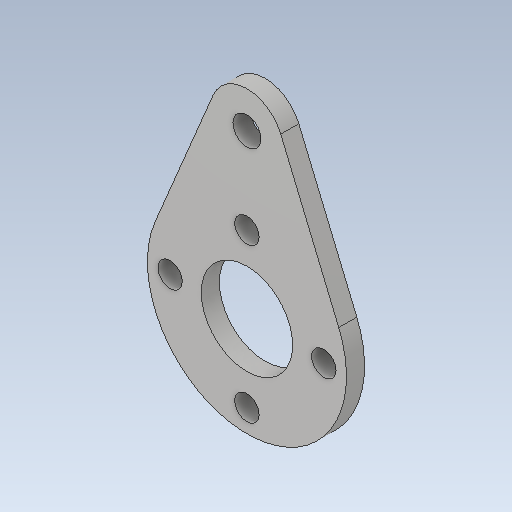
# Autodesk Inventor part: Slider_crank_horn
Saved by Autodesk Inventor 2020.4 (Build 244396000, 396)
## iProperties
Created: 2016-08-24
Part Number: Slider_crank_horn
Material: GFRP
Document SubType Name: Modeling
Designer: hiro
Density: 1.75 g/cm^3
Appearance: 滑らか - 淡い灰色
Mass: 1.33535 g
Surface Area: 10.8308 cm^2
Volume: 0.763059 cm^3
Category: 付け根
Author: hiro
Autodesk Inventor part; units mm, degrees
ref_plane "YZ Plane" through (0, 0, 0) normal (1, 0, 0) x (0, 1, 0)
ref_plane "XZ Plane" through (0, 0, 0) normal (0, 1, 0) x (-1, 0, 0)
ref_plane "XY Plane" through (0, 0, 0) normal (0, 0, 1) x (1, 0, 0)
derived "付け根_基準フレーム_6_1.ipt"
sketch "スケッチ1" plane through (0, 0, 0) normal (0, 0, 1) x (1, 0, 0)
  circle A0 centre (0, 0) radius 11 construction
  circle A1 centre (-13.5, -1) radius 1.35 construction
  line L0 (-13.5, -1) -> (13.5, -1) construction
  line L1 (13.5, -1) -> (13.5, -28) construction
  line L2 (13.5, -28) -> (-13.5, -28) construction
  line L3 (-13.5, -28) -> (-13.5, -1) construction
  circle A2 centre (13.5, -1) radius 1.35 construction
  circle A3 centre (-13.5, -28) radius 1.35 construction
  circle A4 centre (13.5, -28) radius 1.35 construction
  line L4 (0, 18) -> (0, -18) construction
  circle A5 centre (0, -18) radius 7 construction
  line L5 (-12.5, 29.5) -> (-12.5, 24.5) construction
  line L6 (-12.5, 24.5) -> (-7.9564, -18.8342) construction
  line L7 (-12.5, 29.5) -> (12.5, 29.5) construction
  line L8 (12.5, 29.5) -> (12.5, 24.5) construction
  line L9 (12.5, 24.5) -> (7.9564, -18.8342) construction
  arc A6 (-7.9564, -18.8342) -> (7.9564, -18.8342) centre (0, -18) ccw construction
  circle A7 centre (-9.5, 27) radius 1.55 construction
  circle A8 centre (9.5, 27) radius 1.55 construction
  line L10 (-5.51, 27.01) -> (5.51, 27.01) construction
  line L11 (5.51, 27.01) -> (5.51, 24.49) construction
  line L12 (5.51, 24.49) -> (-5.51, 24.49) construction
  line L13 (-5.51, 24.49) -> (-5.51, 27.01) construction
  circle A9 centre (-4.46, 27.01) radius 1.05 construction
  circle A10 centre (-4.46, 24.49) radius 1.05 construction
  circle A11 centre (4.46, 27.01) radius 1.05 construction
  circle A12 centre (4.46, 24.49) radius 1.05 construction
  line L14 (5.5, 27) -> (-5.5, 27) construction
  line L15 (-5.5, 27) -> (-5.5, 24.5) construction
  line L16 (-5.5, 24.5) -> (5.5, 24.5) construction
  line L17 (5.5, 24.5) -> (5.5, 27) construction
  circle A13 centre (0, -18) radius 4.05 construction
  circle A14 centre (0, 8.5) radius 1.35
  circle A15 centre (-8.5, 0) radius 1.35
  circle A16 centre (0, -8.5) radius 1.35
  circle A17 centre (8.5, 0) radius 1.35
  circle A18 centre (0, 0) radius 5.05
  line L18 (-10.147, 4.2472) -> (-3.7359, 19.5638)
  line L19 (3.7359, 19.5638) -> (10.147, 4.2472)
  arc A19 (-10.147, 4.2472) -> (10.147, 4.2472) centre (0, 0) ccw
  arc A20 (3.7359, 19.5638) -> (-3.7359, 19.5638) centre (0, 18) ccw
  circle A21 centre (0, 18) radius 1.55
  line L20 (-10.9545, 1) -> (-14.0575, 1) construction
  line L21 (-14.0575, 1) -> (-24.81, -5.5) construction
  line L22 (-24.81, -5.5) -> (-24.81, -23.5) construction
  line L23 (-24.81, -23.5) -> (-14.0575, -30) construction
  line L24 (-14.0575, -30) -> (14.0575, -30) construction
  line L25 (14.0575, -30) -> (24.81, -23.5) construction
  line L26 (24.81, -23.5) -> (24.81, -5.5) construction
  line L27 (24.81, -5.5) -> (14.0575, 1) construction
  line L28 (14.0575, 1) -> (10.9545, 1) construction
  arc A22 (-10.9545, 1) -> (10.9545, 1) centre (0, 0) ccw construction
  line L29 (-21.76, -10.49) -> (-19.74, -10.49) construction
  line L30 (-19.74, -10.49) -> (-19.74, -18.51) construction
  line L31 (-19.74, -18.51) -> (-21.76, -18.51) construction
  line L32 (-21.76, -18.51) -> (-21.76, -10.49) construction
  line L33 (-19.75, -10.5) -> (-21.75, -10.5) construction
  line L34 (-21.75, -10.5) -> (-21.75, -18.5) construction
  line L35 (-21.75, -18.5) -> (-19.75, -18.5) construction
  line L36 (-19.75, -18.5) -> (-19.75, -10.5) construction
  circle A23 centre (-21.76, -11.54) radius 1.05 construction
  circle A24 centre (-19.74, -11.54) radius 1.05 construction
  circle A25 centre (-19.74, -17.46) radius 1.05 construction
  circle A26 centre (-21.76, -17.46) radius 1.05 construction
  circle A27 centre (-13.5, -1) radius 2 construction
  line L37 (-24.81, -14.5) -> (-19.75, -14.5) construction
  circle A28 centre (-21.76, -11.54) radius 3.05 construction
  circle A29 centre (-13.5, -28) radius 2 construction
  line L38 (21.76, -10.49) -> (19.74, -10.49) construction
  line L39 (19.75, -10.5) -> (21.75, -10.5) construction
  circle A30 centre (19.74, -11.54) radius 1.05 construction
  circle A31 centre (21.76, -11.54) radius 1.05 construction
  circle A32 centre (21.76, -11.54) radius 3.05 construction
  line L40 (24.81, -14.5) -> (19.75, -14.5) construction
  line L41 (19.75, -18.5) -> (19.75, -10.5) construction
  line L42 (21.75, -10.5) -> (21.75, -18.5) construction
  line L43 (19.74, -10.49) -> (19.74, -18.51) construction
  line L44 (21.76, -18.51) -> (21.76, -10.49) construction
  circle A33 centre (19.74, -17.46) radius 1.05 construction
  line L45 (21.75, -18.5) -> (19.75, -18.5) construction
  line L46 (19.74, -18.51) -> (21.76, -18.51) construction
  circle A34 centre (21.76, -17.46) radius 1.05 construction
  line L47 (0, -14.7668) -> (2.8, -16.3834) construction
  line L48 (2.8, -16.3834) -> (2.8, -19.6166) construction
  line L49 (2.8, -19.6166) -> (0, -21.2332) construction
  line L50 (0, -21.2332) -> (-2.8, -19.6166) construction
  line L51 (-2.8, -19.6166) -> (-2.8, -16.3834) construction
  line L52 (-2.8, -16.3834) -> (0, -14.7668) construction
  line L53 (-19.75, 12) -> (19.75, 12) construction
  line L54 (19.75, 12) -> (19.75, -39.5) construction
  line L55 (19.75, -39.5) -> (-19.75, -39.5) construction
  line L56 (-19.75, -39.5) -> (-19.75, 12) construction
  arc A35 (4.1, 18) -> (-4.1, 18) centre (0, 18) ccw construction
  line L57 (-4.1, 18) -> (-4.1, 7.4558) construction
  line L58 (4.1, 18) -> (4.1, 7.4558) construction
  arc A36 (-4.1, 7.4558) -> (4.1, 7.4558) centre (0, 7.4558) ccw construction
  circle A37 centre (0, 18) radius 6.5 construction
  line L59 (-21.75, -2) -> (-19.75, -2) construction
  line L60 (-19.75, -2) -> (-19.75, -27) construction
  line L61 (-19.75, -27) -> (-21.75, -27) construction
  line L62 (-21.75, -27) -> (-21.75, -2) construction
  circle A38 centre (0, -18) radius 36 construction
  line L63 (0, -18) -> (-25.4558, 7.4558) construction
  circle A39 centre (0, 0) radius 18 construction
  line L64 (-18, 0) -> (-25.4558, 7.4558) construction
  point P0 (0, -1)
  point P1 (0, 29.5)
  point P2 (-12.5, 27)
  point P3 (-21.75, -14.5)
extrude "押し出し1" add sketch "スケッチ1" along normal blind 2
